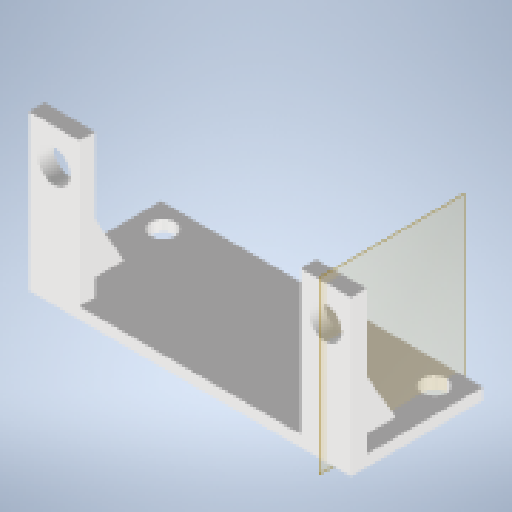
# Autodesk Inventor part: 28BYJ-48_Braket
Saved by Autodesk Inventor 2025.3 (Build 293356000, 356)
## iProperties
Created: 2025-07-13
Part Number: 28BYJ-48_Braket
Material: 一般
Document SubType Name: Modeling
Designer: daisuke
Density: 1 g/cm^3
Appearance: 既定
Author: daisuke
Autodesk Inventor part; units mm, degrees
ref_plane "XZ Plane" through (0, 0, 0) normal (0, 1, 0) x (-1, 0, 0)
ref_plane "XY Plane" through (0, 0, 0) normal (0, 0, 1) x (1, 0, 0)
sketch "スケッチ1" plane through (0, 0, 0) normal (0, 0, 1) x (1, 0, 0)
  line L0 (0, 0) -> (0, 23.3181) construction
  line L1 (-22.6457, 15.5) -> (22.6457, 15.5) construction
  line L2 (-20.3832, 1.5) -> (20.3832, 1.5) construction
  circle A0 centre (0, 15.5) radius 14 construction
  line L3 (-22.6457, 7.5) -> (22.6457, 7.5) construction
  circle A1 centre (-17.5, 15.5) radius 2.1
  circle A2 centre (17.5, 15.5) radius 2.1
  line L4 (-14.25, 20) -> (-20.75, 20)
  line L5 (-20.75, 20) -> (-20.75, 0)
  line L6 (-20.75, 0) -> (-14.25, 0)
  line L7 (-14.25, 0) -> (-14.25, 20)
  line L8 (14.25, 20) -> (20.75, 20)
  line L9 (20.75, 20) -> (20.75, 0)
  line L10 (20.75, 0) -> (14.25, 0)
  line L11 (14.25, 0) -> (14.25, 20)
  line L12 (20.75, 0) -> (20.75, 1.5)
  line L13 (20.75, 1.5) -> (-20.75, 1.5)
  line L14 (-20.75, 1.5) -> (-20.75, 0)
  line L15 (-20.75, 0) -> (20.75, 0)
  point P0 (0, 1.5)
  point P1 (0, 7.5)
  point P2 (-17.5, 20)
  point P3 (17.5, 20)
  point P4 (-14.25, 0)
  point P5 (14.25, 0)
  point P6 (14.25, 1.5)
  point P7 (-14.25, 1.5)
  point P8 (-20.75, 1.5)
  dimension "d0" = 28
  dimension "d1" = 1.5
  dimension "d2" = 8
  dimension "d3" = 4.2
  dimension "d4" = 35
  dimension "d5" = 6.5
  dimension "d6" = 20
  constraints: 32 end point, 9 point on line, 5 midpoint, 5 parallel, 4 horizontal, 3 centre point, 3 perpendicular, 2 collinear, 2 vertical alignment, 1 coincident, 1 equal radius, 1 horizontal alignment, 1 symmetric about line, 1 tangent, 1 vertical
  measures "d0" diameter of A0
  measures "d1" distance from line of L2 L0.start
  measures "d2" distance between parallel lines of L3 L1
  measures "d3" diameter of A1
  measures "d4" distance of A2.centre A1.centre
  measures "d5" distance of L4.start L4.end
  measures "d6" distance of L4.end L5.end
extrude "前" add sketch "スケッチ1" along normal blind 2
extrude "底" add sketch "スケッチ1" against normal blind 15 contours L13 L11 L15 L7 | L7 L6 L5 L13 | L13 L9 L10 L11
ref_plane "作業平面1" through (17.5, 0, 0) normal (1, 0, 0) x (0, 1, 0)
sketch "スケッチ2" plane through (17.5, 0, 0) normal (1, 0, 0) x (0, 1, 0)
  line L0 (11.8923, 0) -> (1.5, -6)
  line L1 (1.5, 0) -> (1.5, -15) projected
  line L2 (1.5, 0) -> (20, 0) projected
  line L3 (11.8923, 0) -> (1.5, 0)
  line L4 (1.5, 0) -> (1.5, -6)
  point P0 (0, 0)
  dimension "d12" = 60
  dimension "d13" = 6
  constraints: 6 end point, 3 point on line, 1 horizontal, 1 perpendicular
  measures "d12" angle of L1 L0
  measures "d13" distance of L0.end L1.start
extrude "リブ" add sketch "スケッチ2" along normal mid plane 2
mirror "ミラー1" about plane through (0, 0, 0) normal (1, 0, 0) of "リブ"
sketch "スケッチ3" plane through (-14.25, 1.5, 2) normal (0, 1, 0) x (1, 0, 0)
  line L0 (14.25, -18.7393) -> (14.25, 26.1406) construction
  line L1 (41.5884, 14) -> (-17.6431, 14) construction
  line L2 (35, 0) -> (28.5, 0) construction
  point P0 (14.25, 2)
  point P1 (31.75, 14)
  point P2 (-3.25, 14)
  dimension "d16" = 35
  dimension "d17" = 14
  constraints: 4 end point, 3 point on line, 1 perpendicular, 1 symmetric about line, 1 vertical
  measures "d16" distance of point (-3.25, 14) point (31.75, 14)
  measures "d17" distance between parallel lines of L1 L2
hole "穴1" at (17.5, 1.5, -12) at (-17.5, 1.5, -12) direction (0, -1, 0) diameter 3.2 end through all
